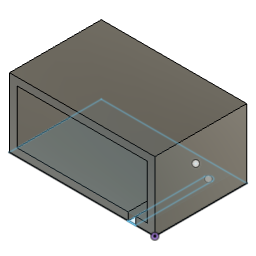
cable_box (Autodesk Fusion 360 design; units mm, degrees)
Autodesk Fusion 360 part; units mm, degrees
sketch "Sketch4" plane through (0, 0, 0) normal (0, 0, 1) x (1, 0, 0)
  line L0 (0, 0) -> (-379.9998, 0)
  line L1 (-379.9998, 0) -> (-379.9998, 239.9997)
  line L2 (-379.9998, 239.9997) -> (0, 239.9997)
  line L3 (0, 239.9997) -> (0, 0)
  constraint horizontal L0
  constraint vertical L1
  constraint horizontal L2
  constraint vertical L3
  constraint coincident L0.start L3.end
extrude "Extrude1" add sketch "Sketch4" along normal blind 180
shell "Shell1" thickness 20 removed faces 1 at (-126.6666, 0, 60)
sketch "Sketch5" plane through (0, 0, 20) normal (0, 0, 1) x (-1, 0, 0)
  line L0 (20, -219.9997) -> (359.9998, -219.9997)
  line L1 (359.9998, -219.9997) -> (359.9998, 0)
  line L2 (359.9998, 0) -> (20, 0)
  line L3 (20, 0) -> (20, -219.9997)
  arc A0 (91.5155, -197.8612) -> (90.4492, -197.9194) centre (90.9821, -197.8846) ccw
sketch "Sketch6" plane through (0, 0, 0) normal (0, 0, 1) x (1, 0, 0)
  line L0 (-49.7545, -0.5052) -> (-49.7545, 199.4948)
  arc A0 (-49.7545, 199.4948) -> (-69.7394, 199.4948) centre (-59.7469, 199.4948) ccw
  line L1 (-69.7394, 199.4948) -> (-69.7394, -0.4848)
  line L2 (-69.7394, -0.4848) -> (-49.7545, -0.5052)
  dimension "d5" = 200
  constraint vertical L0
  constraint tangent L0 A0
  constraint tangent A0 L1
  constraint vertical L1
  measures "d5" distance of L0.start L0.end
extrude "Extrude2" cut sketch "Sketch6" along normal blind 20
